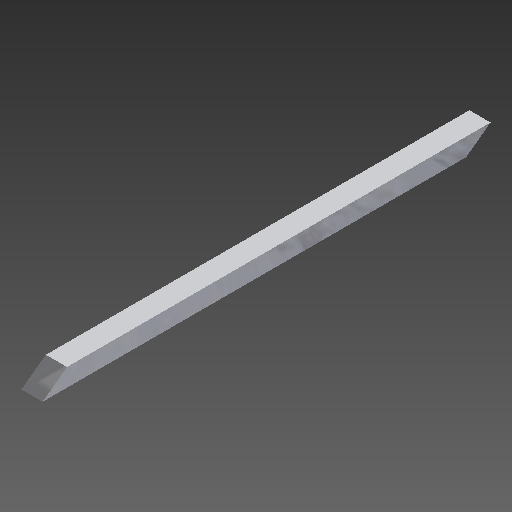
# Autodesk Inventor part: 3d_Welding_Tooling - Acetal Stick
Saved by Autodesk Inventor 2018.3 (Build 223284000, 284)
## iProperties
Created: 2026-01-26
Part Number: 3d_Welding_Tooling - Acetal Stick
Material: Acetal Resin, White
Document SubType Name: Modeling
Designer: aca6
Density: 1.425 g/cm^3
Appearance: Smooth - White
Manufacturer-1: {"Name": "Hanstar Technologies Co., Ltd", "PartNumber": "3d_Welding_Tooling - Acetal Stick", "Link": ""}
Manufacturer-2: {"Name": "SHENZHEN JINYIHE PROTOTYPE TECHNOLOGIES CO., LTD", "PartNumber": "3d_Welding_Tooling - Acetal Stick", "Link": ""}
Manufacturer-3: {"Name": "Shenzhen city Xavier Precision Co., Ltd.", "PartNumber": "3d_Welding_Tooling - Acetal Stick", "Link": ""}
Manufacturer-4: {"Name": "", "PartNumber": "", "Link": ""}
Manufacturer-5: {"Name": "", "PartNumber": "", "Link": ""}
Provider-1: {"Name": "", "PartNumber": "", "Link": ""}
Provider-2: {"Name": "", "PartNumber": "", "Link": ""}
Provider-3: {"Name": "", "PartNumber": "", "Link": ""}
Provider-4: {"Name": "", "PartNumber": "", "Link": ""}
Provider-5: {"Name": "", "PartNumber": "", "Link": ""}
Author: aca6
Comments: DIN-ISO-2768-mK
Autodesk Inventor part; units mm, degrees
ref_plane "YZ Plane" through (0, 0, 0) normal (1, 0, 0) x (0, 1, 0)
ref_plane "XZ Plane" through (0, 0, 0) normal (0, 1, 0) x (-1, 0, 0)
ref_plane "XY Plane" through (0, 0, 0) normal (0, 0, 1) x (1, 0, 0)
sketch "Sketch1" plane through (0, 0, 0) normal (0, 0, 1) x (1, 0, 0)
  line L0 (1, -7.5) -> (-4, -7.5)
  line L1 (-4, -7.5) -> (1.7735, 2.5)
  line L2 (1, -7.5) -> (6.7735, 2.5)
  line L3 (1.7735, 2.5) -> (6.7735, 2.5)
  line L4 (0, 0) -> (1.5241, 0) construction
  line L5 (0, 0) -> (0, 2.8469) construction
  dimension "d1" = 60
  dimension "d2" = 120
  dimension "d4" = 5
  dimension "d6" = 5
  dimension "d7" = 10
  dimension "d8" = 2.5
  dimension "d9" = 4
  constraints: 12 end point, 3 horizontal, 2 vertical, 1 other
  measures "d1" angle of L0 L1
  measures "d2" angle of L0 L2
  measures "d4" distance of L0.start L0.end
  measures "d6" distance of L1.end L2.end
  measures "d7" vertical distance of L0.start L2.end
  measures "d8" distance between parallel lines of L3 L4
  measures "d9" distance from line of L5 L0.end
extrude "Extrusion1" add sketch "Sketch1" along normal blind 100
body "Solid1"
